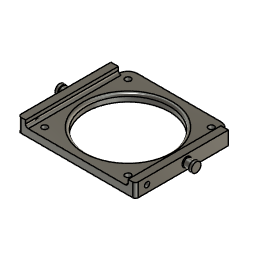
FS80 Unified Adapter v11 (Autodesk Fusion 360 design; units mm, degrees)
Autodesk Fusion 360 part; units mm, degrees
sketch "Schizzo1" plane through (0, 0, 0) normal (0, 0, 1) x (1, 0, 0)
  line L0 (-35.999, 68.9836) -> (39.201, 68.9836)
  line L1 (39.201, 68.9836) -> (39.201, -6.0164)
  line L2 (39.201, -6.0164) -> (-35.999, -6.0164)
  line L3 (-35.999, -6.0164) -> (-35.999, 68.9836)
  line L4 (-35.999, 31.4836) -> (39.201, 31.4836) construction
  line L5 (1.601, 68.9836) -> (1.601, -6.0164) construction
  circle A0 centre (1.601, 31.4836) radius 30.5
  line L6 (32.101, 0.9836) -> (-28.899, 0.9836) construction
  line L7 (-28.899, 0.9836) -> (-28.899, 61.9836) construction
  line L8 (-28.899, 61.9836) -> (32.101, 61.9836) construction
  line L9 (32.101, 61.9836) -> (32.101, 0.9836) construction
  line L10 (32.101, 0.9836) -> (-28.899, 61.9836) construction
  line L11 (-28.899, 0.9836) -> (32.101, 61.9836) construction
  circle A1 centre (-28.899, 61.9836) radius 2.1
  circle A2 centre (32.101, 61.9836) radius 2.1
  circle A3 centre (32.101, 0.9836) radius 2.1
  circle A4 centre (32.201, 61.9836) radius 7
  circle A5 centre (-28.899, 0.9836) radius 2.1
  line L12 (-41.399, 61.9836) -> (-35.999, 61.9836)
  line L13 (-35.999, 61.9836) -> (-35.999, 0.9836)
  line L14 (-35.999, 0.9836) -> (-41.399, 0.9836)
  line L15 (-41.399, 0.9836) -> (-41.399, 61.9836)
  line L16 (44.601, 61.9836) -> (39.201, 61.9836)
  line L17 (44.601, 0.9836) -> (44.601, 61.9836)
  line L18 (39.201, 61.9836) -> (39.201, 0.9836)
  line L19 (39.201, 0.9836) -> (44.601, 0.9836)
  circle A6 centre (-28.899, 61.9836) radius 3.6
  circle A7 centre (32.101, 61.9836) radius 3.6
  circle A8 centre (-28.899, 0.9836) radius 3.6
  circle A9 centre (32.101, 0.9836) radius 3.6
  line L20 (-41.399, 0.9836) -> (-35.999, 0.9836)
  line L21 (-35.999, 0.9836) -> (-35.999, -6.0164)
  line L22 (-35.999, -6.0164) -> (-41.399, -6.0164)
  line L23 (-41.399, -6.0164) -> (-41.399, 0.9836)
  line L24 (44.601, 0.9836) -> (39.201, 0.9836)
  line L25 (39.201, 0.9836) -> (39.201, -6.0164)
  line L26 (39.201, -6.0164) -> (44.601, -6.0164)
  line L27 (44.601, -6.0164) -> (44.601, 0.9836)
  circle A10 centre (-28.999, 61.9836) radius 7
  point P0 (1.601, 31.4836)
  point P1 (-28.899, 0.9836)
  dimension "d1" = 75.2
  dimension "d2" = 75
  dimension "d3" = 61
  dimension "d4" = 61
  dimension "d5" = 61
  dimension "d6" = 4.2
  dimension "d8" = 7
  dimension "d13" = 5.4
  dimension "d22" = 7.2
  dimension "d60" = 7
  dimension "d70" = 86
  constraint horizontal L0
  constraint vertical L1
  constraint horizontal L2
  constraint vertical L3
  constraint midpoint L3 L4.start
  constraint midpoint L1 L4.end
  constraint midpoint L0 L5.start
  constraint midpoint L2 L5.end
  constraint midpoint L4 P0
  constraint horizontal L6
  constraint perpendicular L6 L7
  constraint parallel L6 L8
  constraint parallel L7 L9
  constraint coincident L10 P0
  constraint coincident L11 P0
  constraint coincident P0 A0.centre
  constraint coincident L7.end L8.start
  constraint symmetric L5 A1 A2
  constraint symmetric L4 L7.end P1
  constraint symmetric L4 A2 A3
  constraint tangent L0 A4
  constraint tangent L1 A4
  constraint symmetric L4 A1 A5
  constraint horizontal L12
  constraint vertical L13
  constraint horizontal L14
  constraint vertical L15
  constraint collinear L8 L12
  constraint collinear L3 L13
  constraint collinear L6 L14
  constraint symmetric L5 L12.start L16.start
  constraint symmetric L5 L12.end L16.end
  constraint symmetric L5 L13.end L18.end
  constraint symmetric L5 L14.end L17.start
  constraint concentric A1 A6
  constraint symmetric L5 A6 A7
  constraint symmetric L4 A6 A8
  constraint symmetric L4 A7 A9
  constraint horizontal L20
  constraint vertical L21
  constraint horizontal L22
  constraint vertical L23
  constraint horizontal L24
  constraint vertical L25
  constraint horizontal L26
  constraint vertical L27
  constraint tangent L0 A10
  constraint tangent L3 A10
  measures "d1" distance of L0.start L0.end
  measures "d2" distance of L0.start L2.end
  measures "d3" diameter of A0
  measures "d4" distance of L7.end L8.end
  measures "d5" distance of P1 L7.end
  measures "d6" diameter of A1
  measures "d8" radius of A4
  measures "d13" distance of L13 L15
  measures "d22" diameter of A6
  measures "d60" radius of A10
  measures "d70" distance of L15 L17
extrude "Estrusione1" add sketch "Schizzo1" along normal blind 5.5 contours L0 L1 L2 L3 A4 L13 L18 L21 L25 A10 | A10 | A4 | A6 | A7 | A8 | A9
extrude "Estrusione2" add sketch "Schizzo1" along normal blind 10 contours L3 L12 L13 L14 L15 L20 | L3 L14 L20 L21 L22 L23 | L1 L16 L17 L18 L19 L24 | L1 L19 L24 L25 L26 L27
fillet "Raccordo1" radius 2 1 edges at (39.201, 27.9836, 5.5)
fillet "Raccordo1" radius 2 1 edges at (-35.999, 27.9836, 5.5)
sketch "Schizzo2" plane through (-41.399, 0, 0) normal (-1, 0, 0) x (0, -1, 0)
  line L0 (-61.9836, 0) -> (6.0164, 0)
  line L1 (6.0164, 10) -> (-61.9836, 10)
  line L2 (-61.9836, 10) -> (-61.9836, 0)
  line L3 (-61.9836, 10) -> (-4.3362, 10) construction
  line L4 (-4.3362, 10) -> (-4.3362, 0) construction
  line L5 (-4.3362, 0) -> (-61.9836, 0) construction
  line L6 (-61.9836, 0) -> (-61.9836, 10) construction
  line L7 (-0.9836, 0) -> (-61.9836, 0) construction
  line L8 (-61.9836, 5) -> (-4.3362, 5) construction
  circle A0 centre (-31.4836, 4.765) radius 2.9
  circle A1 centre (-31.4836, 4.765) radius 3.5
  line L9 (6.0164, 0) -> (6.0164, 10)
  circle A2 centre (-2.4846, 5) radius 1.9
  dimension "d25" = 10
  dimension "d27" = 5.8
  dimension "d28" = 7
  dimension "d56" = 3.8
  dimension "d64" = 30.5
  dimension "d65" = 29
  constraint horizontal L3
  constraint vertical L4
  constraint horizontal L5
  constraint vertical L6
  constraint coincident L1.end L2.start
  constraint collinear L5 L7
  constraint midpoint L6 L8.start
  constraint midpoint L4 L8.end
  constraint coincident L8 A2.centre
  constraint coincident A0.centre A1.centre
  measures "d25" distance of L3 L7
  measures "d27" diameter of A0
  measures "d28" diameter of A1
  measures "d56" diameter of A2
  measures "d64" distance of L6 A0.centre
  measures "d65" distance of A0.centre A2.centre
extrude "Estrusione4" add sketch "Schizzo2" along normal blind 7 contours A0
extrude "Estrusione5" add sketch "Schizzo2" against normal blind 2 from surface at 7 contours A1
fillet "Raccordo4" radius 0.5 1 edges at (-41.399, 34.1874, 5.8137)
extrude "Estrusione10" cut sketch "Schizzo2" against normal up to surface (5.4 mm away) contours A2
sketch "Schizzo3" plane through (44.601, 0, 0) normal (1, 0, 0) x (0, 1, 0)
  line L0 (-6.0164, 0) -> (61.9836, 0)
  line L1 (61.9836, 0) -> (61.9836, 10)
  line L2 (61.9836, 10) -> (-6.0164, 10)
  line L3 (0.9836, 10) -> (61.9836, 10) construction
  line L4 (61.9836, 10) -> (61.9836, 0) construction
  line L5 (61.9836, 0) -> (0.9836, 0) construction
  line L6 (0.9836, 0) -> (0.9836, 10) construction
  line L7 (0.9836, 0) -> (61.9836, 0) construction
  line L8 (0.9836, 5) -> (61.9836, 5) construction
  circle A0 centre (31.4836, 5) radius 2.9
  circle A1 centre (31.4836, 5) radius 3.5
  line L9 (-6.0164, 10) -> (-6.0164, 0)
  circle A2 centre (2.4836, 5) radius 1.9
  dimension "d36" = 5.8
  dimension "d37" = 7
  dimension "d49" = 3.8
  dimension "d50" = 29
  dimension "d51" = 30.5
  constraint horizontal L3
  constraint vertical L4
  constraint horizontal L5
  constraint vertical L6
  constraint collinear L5 L7
  constraint collinear L2 L3
  constraint collinear L1 L4
  constraint midpoint L6 L8.start
  constraint midpoint L4 L8.end
  constraint concentric A0 A1
  constraint coincident L8 A2.centre
  measures "d36" diameter of A0
  measures "d37" diameter of A1
  measures "d49" diameter of A2
  measures "d50" distance of A0.centre A2.centre
  measures "d51" distance of L4 A0.centre
extrude "Estrusione6" add sketch "Schizzo3" along normal blind 7 contours A0
extrude "Estrusione7" add sketch "Schizzo3" against normal blind 2 from surface at 7 contours A1
fillet "Raccordo5" radius 0.5 1 edges at (44.601, 28.7799, 6.0487)
extrude "Estrusione11" cut sketch "Schizzo3" against normal up to surface (5.4 mm away) contours A2
fillet "Raccordo6" radius 2 1 edges at (-41.399, -6.0164, 5)
fillet "Raccordo6" radius 2 1 edges at (44.601, -6.0164, 5)
fillet "Raccordo7" radius 2 1 edges at (-26.835, 42.5129, 5.5)
equation "d1 = 75 mm + 0.2 mm"
equation "d51 = ( 61 / 2 ) * 1 mm"
equation "d64 = ( 61 / 2 ) * 1 mm"
